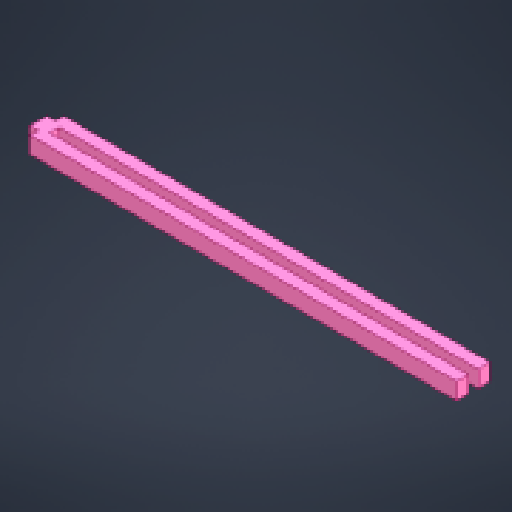
# Autodesk Inventor part: Widełki
Saved by Autodesk Inventor 2023 (Build 270158000, 158)
## iProperties
Created: 2023-05-08
Part Number: Widełki
Material: Generic
Document SubType Name: Modeling
Designer: szykr
Density: 1 g/cm^3
Appearance: Pink
Author: szykr
Autodesk Inventor part; units mm, degrees
ref_plane "YZ Plane" through (0, 0, 0) normal (1, 0, 0) x (0, 1, 0)
ref_plane "XZ Plane" through (0, 0, 0) normal (0, 1, 0) x (-1, 0, 0)
ref_plane "XY Plane" through (0, 0, 0) normal (0, 0, 1) x (1, 0, 0)
sketch "Sketch1" plane through (0, 0, 0) normal (0, 1, 0) x (-1, 0, 0)
  line L0 (2.9, 0) -> (2.9, -3) projected
  line L1 (1.5, 0) -> (2.9, 0) projected
  line L2 (1.5, 1.4) -> (1.5, 0) projected
  line L3 (0, 1.4) -> (1.5, 1.4) projected
  line L4 (0, -4.4) -> (0, 1.4) projected
  line L5 (1.5, -4.4) -> (0, -4.4) projected
  line L6 (1.5, -3) -> (1.5, -4.4) projected
  line L7 (1.5, -3) -> (2.9, -3) projected
  line L8 (0.1, -4.3) -> (0.1, 1.3)
  line L9 (0.1, 1.3) -> (1.4, 1.3)
  line L10 (1.4, 1.3) -> (1.4, -0.1)
  line L11 (1.4, -0.1) -> (2.8, -0.1)
  line L12 (2.8, -0.1) -> (2.8, -2.9)
  line L13 (2.8, -2.9) -> (1.4, -2.9)
  line L14 (1.4, -2.9) -> (1.4, -4.3)
  line L15 (1.4, -4.3) -> (0.1, -4.3)
  line L16 (0.1, -4.3) -> (-69.9, -4.3)
  line L17 (-69.9, -4.3) -> (-69.9, -2.3)
  line L18 (-69.9, -2.3) -> (0.1, -2.3)
  line L19 (0.1, -2.3) -> (0.1, -4.3)
  line L20 (0.1, 1.3) -> (-69.9, 1.3)
  line L21 (-69.9, 1.3) -> (-69.9, -0.7)
  line L22 (-69.9, -0.7) -> (0.1, -0.7)
  line L23 (0.1, -0.7) -> (0.1, 1.3)
  point P0 (0, 0)
  point P1 (0.1, -0.7)
  point P2 (0.1, -2.3)
  dimension "d0" = 0.1
  dimension "d1" = 1.6
  dimension "d2" = 70
  constraints: 32 end point, 4 parallel, 2 equal length, 2 horizontal, 2 perpendicular, 7 other
  measures "d0" distance between parallel lines of L5 L15
  measures "d1" distance between parallel lines of L18 L22
  measures "d2" distance between parallel lines of L19 L17
extrude "Extrusion1" add sketch "Sketch1" along normal blind 2.8 contours L20 L8 L22 L4 | L4 L22 L21 L20 | L16 L17 L18 L4 | L4 L18 L8 L16 | L9 L10 L11 L12 L13 L14 L15 L8
equation "\"d0\" = slack"
equation "\"slack\" = 0.1"
equation "\"slack2\" = 0.1"
body "Solid1"
